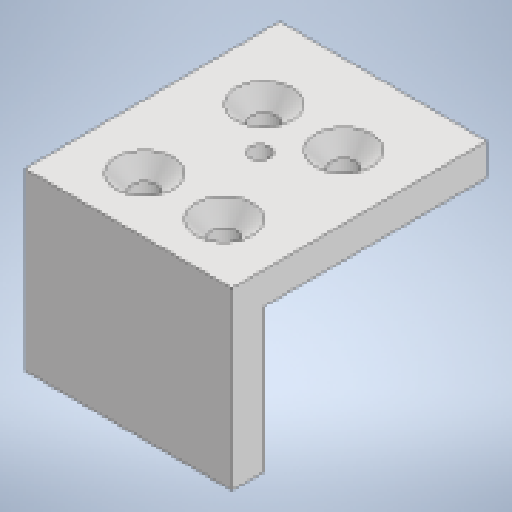
# Autodesk Inventor part: grantry_holder_R
Saved by Autodesk Inventor 2024.1 (Build 281209000, 209)
## iProperties
Created: 2023-10-02
Part Number: grantry_holder_R
Material: Generic
Document SubType Name: Modeling
Designer: l1534
Density: 1 g/cm^3
Appearance: Default
Author: l1534
Autodesk Inventor part; units mm, degrees
ref_plane "YZ Plane" through (0, 0, 0) normal (1, 0, 0) x (0, 1, 0)
ref_plane "XZ Plane" through (0, 0, 0) normal (0, 1, 0) x (-1, 0, 0)
ref_plane "XY Plane" through (0, 0, 0) normal (0, 0, 1) x (1, 0, 0)
sketch "Sketch1" plane through (0, 0, 0) normal (0, 1, 0) x (-1, 0, 0)
  line L0 (13.2828, -12.6642) -> (-12.7172, -12.6642)
  line L1 (-12.7172, -12.6642) -> (-12.7172, 17.3358)
  line L2 (-12.7172, 17.3358) -> (13.2828, 17.3358)
  line L3 (13.2828, 17.3358) -> (13.2828, -12.6642)
  point P0 (0, 0)
  dimension "d0" = 26
  dimension "d1" = 30
  constraints: 8 end point, 2 parallel, 1 horizontal, 1 perpendicular
  measures "d0" distance of L0.start L0.end
  measures "d1" distance of L0.end L1.end
extrude "Extrusion1" add sketch "Sketch1" along normal blind 4
sketch "Sketch2" plane through (0, 4, 0) normal (0, 1, 0) x (1, 0, 0)
  circle A0 centre (-5.2828, 2.6642) radius 1.55
  circle A1 centre (4.7172, 2.6642) radius 1.55
  circle A2 centre (-5.2828, -12.3358) radius 1.55
  circle A3 centre (4.7172, -12.3358) radius 1.55
  line L0 (-13.2828, -17.3358) -> (12.7172, -17.3358) projected
  line L1 (-13.2828, 12.6642) -> (-13.2828, -17.3358) projected
  point P0 (0, 0)
  dimension "d4" = 3.1
  dimension "d5" = 3.1
  dimension "d6" = 3.1
  dimension "d7" = 3.1
  dimension "d8" = 10
  dimension "d9" = 10
  dimension "d10" = 15
  dimension "d11" = 15
  dimension "d12" = 5
  dimension "d13" = 5
  dimension "d14" = 8
  dimension "d15" = 8
  constraints: 4 centre point
  measures "d4" diameter of A0
  measures "d5" diameter of A1
  measures "d6" diameter of A2
  measures "d7" diameter of A3
  measures "d8" distance of A0.centre A1.centre
  measures "d9" distance of A2.centre A3.centre
  measures "d10" distance of A3.centre A1.centre
  measures "d11" distance of A2.centre A0.centre
  measures "d12" distance from line of L0 A2.centre
  measures "d13" distance from line of L0 A3.centre
  measures "d14" distance from line of L1 A0.centre
  measures "d15" distance from line of L1 A2.centre
extrude "Extrusion2" cut sketch "Sketch2" against normal through all
sketch "Sketch3" plane through (0, 0, 0) normal (0, -1, 0) x (1, 0, 0)
  point P0 (0, 0)
sketch "Sketch4" plane through (-13.2828, 0, -12.6642) normal (-1, 0, 0) x (0, 0, 1)
  line L0 (30, 4) -> (0, 4) projected
  line L1 (28, 4) -> (32, 4)
  line L2 (32, 4) -> (32, -18)
  line L3 (32, -18) -> (28, -18)
  line L4 (28, -18) -> (28, 4)
  line L5 (30, 0) -> (30, 4) projected
  point P0 (12.6642, 0)
  dimension "d18" = 2
  dimension "d19" = 4
  dimension "d20" = 22
  constraints: 8 end point, 2 parallel, 1 horizontal, 1 perpendicular, 1 point on line
  measures "d18" distance between parallel lines of L5 L4
  measures "d19" distance of L1.start L1.end
  measures "d20" distance of L1.end L2.end
extrude "Extrusion3" add sketch "Sketch4" against normal up to surface (26 mm away)
chamfer "Chamfer1" distance 2 angle 45 4 edges at (-6.8328, 4, 12.3358) (3.1672, 4, 12.3358) (-6.8328, 4, -2.6642) (3.1672, 4, -2.6642)
sketch "Sketch5" plane through (0, 4, 0) normal (0, 1, 0) x (1, 0, 0)
  circle A0 centre (-0.2828, -2.8358) radius 1.25
  line L0 (12.7172, 12.6642) -> (-13.2828, 12.6642) projected
  line L1 (-13.2828, 12.6642) -> (-13.2828, -19.3358) projected
  point P0 (0, 0)
  dimension "d26" = 2.5
  dimension "d27" = 15.5
  dimension "d28" = 13
  constraints: 1 centre point
  measures "d26" diameter of A0
  measures "d27" distance from line of L0 A0.centre
  measures "d28" distance from line of L1 A0.centre
extrude "Extrusion4" cut sketch "Sketch5" against normal through all
sketch "Sketch6" plane through (0, 0, 0) normal (0, -1, 0) x (1, 0, 0)
  line L0 (12.7172, -12.6642) -> (-13.2828, -12.6642) projected
  line L1 (-13.2828, -12.6642) -> (12.7172, -12.6642)
  line L2 (12.7172, -12.6642) -> (12.7172, -7.6642)
  line L3 (12.7172, -7.6642) -> (-13.2828, -7.6642)
  line L4 (-13.2828, -7.6642) -> (-13.2828, -12.6642)
  point P0 (0, 0)
  dimension "d31" = 5
  constraints: 8 end point, 2 parallel, 1 horizontal, 1 perpendicular
  measures "d31" distance of L3.end L0.end
extrude "Extrusion5" add sketch "Sketch6" along normal blind 25
body "Solid1"
